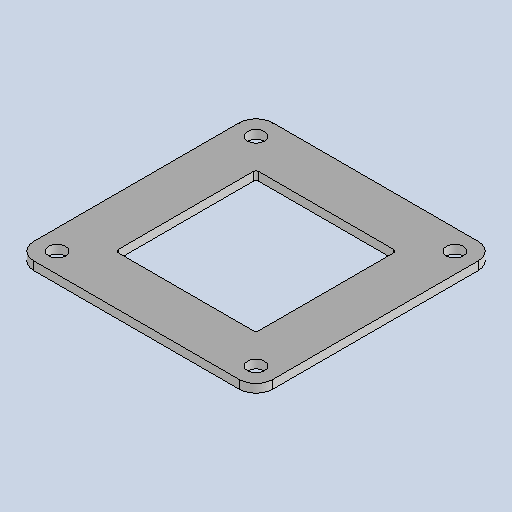
# Autodesk Inventor part: TKS 3525 FDS Way FLANGE
Saved by Autodesk Inventor 2025 (Build 290162010, 162A)
## iProperties
Created: 2025-06-24
Part Number: TKS 3525 FDS Way FLANGE
Material: Stainless Steel
Document SubType Name: Sheet Metal
Designer: user
Mass: 103.446 g
Surface Area: 101.897 cm^2
Volume: 12.9307 cm^3
Density: 8 g/cm^3
Sheet Metal Rule: AISI304 2mm Die16
Sheet Metal Width: 85,000 mm
Sheet Metal Length: 85,000 mm
Sheet Metal Area: 7225,000 mm^2
Appearance: Default
Flat Pattern Width: 8.5 cm
Flat Pattern Length: 8.5 cm
Flat Pattern Area: 72.25 cm^2
Author: user
Autodesk Inventor part; units mm, degrees
ref_plane "YZ Plane" through (0, 0, 0) normal (1, 0, 0) x (0, 1, 0)
ref_plane "XZ Plane" through (0, 0, 0) normal (0, 1, 0) x (-1, 0, 0)
ref_plane "XY Plane" through (0, 0, 0) normal (0, 0, 1) x (1, 0, 0)
sketch "Sketch1" plane through (0, 0, 0) normal (0, 0, 1) x (1, 0, 0)
  line L0 (-42.5, -42.5) -> (42.5, -42.5)
  line L1 (42.5, -42.5) -> (42.5, 42.5)
  line L2 (42.5, 42.5) -> (-42.5, 42.5)
  line L3 (-42.5, 42.5) -> (-42.5, -42.5)
  line L4 (-42.5, -42.5) -> (42.5, 42.5) construction
  line L5 (42.5, -42.5) -> (-42.5, 42.5) construction
  line L6 (25, -25) -> (-25, -25)
  line L7 (-25, -25) -> (-25, 25)
  line L8 (-25, 25) -> (25, 25)
  line L9 (25, 25) -> (25, -25)
  line L10 (25, -25) -> (-25, 25) construction
  line L11 (-25, -25) -> (25, 25) construction
  point P0 (0, 0)
  dimension "d154" = 85
  dimension "d155" = 85
  dimension "d172" = 50
  measures "d154" distance of L1.end L2.end
  measures "d155" distance of L0.end L1.end
  measures "d172" distance of L7.end L8.end
extrude "Plate5" add sketch "Sketch1" along normal blind 3
sketch "Sketch9" plane through (0, 0, 3) normal (0, 0, 1) x (1, 0, 0)
  circle A0 centre (35.3553, -35.3553) radius 3
  line L0 (35.3553, 35.3553) -> (-35.3553, 35.3553) construction
  line L1 (-35.3553, 35.3553) -> (-35.3553, -35.3553) construction
  line L2 (-35.3553, -35.3553) -> (35.3553, -35.3553) construction
  line L3 (35.3553, -35.3553) -> (35.3553, 35.3553) construction
  line L4 (35.3553, 35.3553) -> (-35.3553, -35.3553) construction
  line L5 (-35.3553, 35.3553) -> (35.3553, -35.3553) construction
  circle A1 centre (-35.3553, -35.3553) radius 3
  circle A2 centre (35.3553, 35.3553) radius 3
  circle A3 centre (-35.3553, 35.3553) radius 3
  circle A4 centre (0, 0) radius 50 construction
  dimension "d180" = 100
  dimension "d174" = 6
  constraints: 12 end point, 8 coincident, 4 centre point, 3 equal radius, 2 midpoint, 2 parallel, 2 perpendicular, 1 horizontal, 3 other
  measures "d174" diameter of A0
extrude "Cut2" cut sketch "Sketch9" against normal blind 3
fillet "Corner Round1" radius 6 4 edges at (42.5, 42.5, 1.5) (-42.5, 42.5, 1.5) (-42.5, -42.5, 1.5) (42.5, -42.5, 1.5)
fillet "Corner Round2" radius 1 4 edges at (-25, 25, 1.5) (-25, -25, 1.5) (25, -25, 1.5) (25, 25, 1.5)
body "Solid3"
